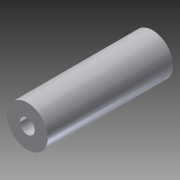
# Autodesk Inventor part: Coupling Bushing
Saved by Autodesk Inventor 2013 (Build 170138000, 138)
## iProperties
Created: 2014-08-02
Part Number: Coupling Bushing
Material: ABS Plastic
Document SubType Name: Modeling
Designer: Kyle
Density: 1 g/cm^3
Author: Kyle
Autodesk Inventor part; units mm, degrees
ref_plane "YZ Plane" through (0, 0, 0) normal (1, 0, 0) x (0, 1, 0)
ref_plane "XZ Plane" through (0, 0, 0) normal (0, 1, 0) x (-1, 0, 0)
ref_plane "XY Plane" through (0, 0, 0) normal (0, 0, 1) x (1, 0, 0)
sketch "Sketch1" plane through (0, 0, 0) normal (0, 0, 1) x (1, 0, 0)
  arc A0 (-0.9144, -1.2192) -> (-0.9144, 1.2192) centre (0, 0) ccw
  line L0 (-0.9144, 1.2192) -> (-0.9144, -1.2192)
  circle A1 centre (0, 0) radius 4.7625
  point P0 (-0.889, 0)
  point P1 (1.524, 0)
  dimension "d0" = 3.048
  dimension "d2" = 2.413
  dimension "d3" = 9.525
  constraints: 3 point on circle, 2 centre point, 2 coincident, 2 end point, 1 vertical
  measures "d0" diameter of A0
  measures "d2" distance of point (-0.889, 0) point (1.524, 0)
  measures "d3" diameter of A1
extrude "Extrusion1" add sketch "Sketch1" along normal blind 10.16
sketch "Sketch2" plane through (0, 0, 10.16) normal (0, 0, 1) x (1, 0, 0)
  circle A0 centre (0, 0) radius 4.7625 projected
extrude "Extrusion2" add sketch "Sketch2" along normal blind 6.35
sketch "Sketch3" plane through (0, 0, 16.51) normal (0, 0, 1) x (1, 0, 0)
  circle A0 centre (0, 0) radius 4.7625 projected
  circle A1 centre (0, 0) radius 1.7145
  dimension "d8" = 3.429
  constraints: 1 centre point, 1 coincident
  measures "d8" diameter of A1
extrude "Extrusion3" add sketch "Sketch3" along normal blind 12.7
body "Solid1"
